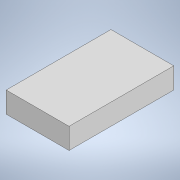
# Autodesk Inventor part: middlebit
Saved by Autodesk Inventor 2020.1 (Build 241239000, 239)
## iProperties
Created: 2019-12-06
Part Number: middlebit
Material: Generic
Document SubType Name: Modeling
Designer: tbloo
Density: 1 g/cm^3
Appearance: Default
Author: tbloo
Autodesk Inventor part; units mm, degrees
ref_plane "YZ Plane" through (0, 0, 0) normal (1, 0, 0) x (0, 1, 0)
ref_plane "XZ Plane" through (0, 0, 0) normal (0, 1, 0) x (-1, 0, 0)
ref_plane "XY Plane" through (0, 0, 0) normal (0, 0, 1) x (1, 0, 0)
sketch "Sketch1" plane through (0, 0, 0) normal (0, 1, 0) x (-1, 0, 0)
  line L0 (0, 0) -> (96, 0)
  line L1 (96, 0) -> (96, 160)
  line L2 (96, 160) -> (0, 160)
  line L3 (0, 160) -> (0, 0)
  dimension "d0" = 96
  dimension "d1" = 160
  constraints: 8 end point, 2 parallel, 1 horizontal, 1 perpendicular
  measures "d0" distance of L2.end L1.end
  measures "d1" distance of L1.end L0.end
extrude "Extrusion1" add sketch "Sketch1" along normal blind 32
body "Solid1"
